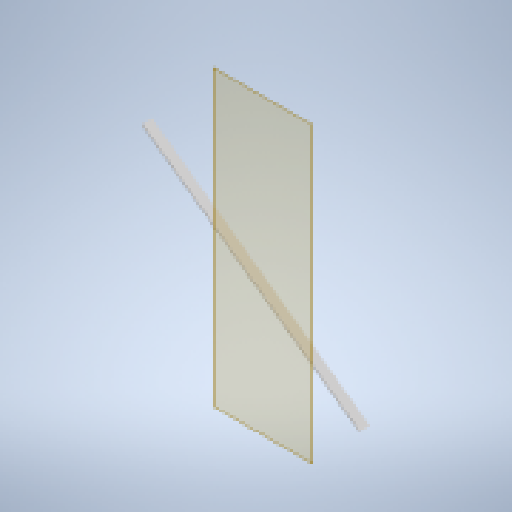
# Autodesk Inventor part: Soportes
Saved by Autodesk Inventor 2024 (Build 280153000, 153)
## iProperties
Created: 2023-08-17
Part Number: Soportes
Material: Genérico
Document SubType Name: Modeling
Designer: sergi
Density: 1 g/cm^3
Appearance: Valor por defecto
Author: sergi
Autodesk Inventor part; units mm, degrees
ref_plane "YZ Plane" through (0, 0, 0) normal (1, 0, 0) x (0, 1, 0)
ref_plane "XZ Plane" through (0, 0, 0) normal (0, 1, 0) x (-1, 0, 0)
ref_plane "XY Plane" through (0, 0, 0) normal (0, 0, 1) x (1, 0, 0)
ref_plane "Plano de trabajo1" through (0, 0, 0) normal (0, 0, 1) x (1, 0, 0)
sketch "Boceto1" plane through (0, 0, 0) normal (0, 0, 1) x (1, 0, 0)
  line L0 (-46.3948, 33.5716) -> (-52.5431, 31.0384) projected
  line L1 (-45.911, 40.2037) -> (-46.3948, 33.5716) projected
  line L2 (-128.559, 100.0083) -> (-45.911, 40.2037) projected
  line L3 (-134.7073, 97.4751) -> (-128.559, 100.0083) projected
  line L4 (-135.1911, 90.843) -> (-134.7073, 97.4751) projected
  line L5 (-52.5431, 31.0384) -> (-135.1911, 90.843) projected
  line L6 (-127.1601, 101.9415) -> (-44.5121, 42.1369) projected
  line L7 (-126.3896, 103.0063) -> (-43.7416, 43.2017) projected
  line L8 (-53.942, 29.1052) -> (-136.59, 88.9098) projected
  line L9 (-137.3604, 87.845) -> (-136.59, 88.9098) projected
  line L10 (-54.7125, 28.0404) -> (-137.3604, 87.845) projected
  line L11 (-126.3896, 103.0063) -> (-127.1601, 101.9415) projected
  line L12 (-136.0968, 89.5913) -> (-53.4489, 29.7866) projected
  line L13 (-45.0053, 41.4554) -> (-127.6532, 101.2601) projected
  line L14 (-127.1601, 101.9415) -> (-131.5092, 100.8886) projected
  line L15 (-136.0968, 89.5913) -> (-135.1911, 90.843) projected
  line L16 (-127.6532, 101.2601) -> (-128.559, 100.0083) projected
  line L17 (-136.59, 88.9098) -> (-136.9497, 93.3701) projected
  line L18 (-136.59, 88.9098) -> (-136.9497, 93.3701) projected
  line L19 (-53.942, 29.1052) -> (-136.59, 88.9098) projected
  line L20 (-49.5929, 30.1581) -> (-53.942, 29.1052) projected
  line L21 (-49.5929, 30.1581) -> (-136.9497, 93.3701) projected
  line L22 (-136.0968, 89.5913) -> (-136.6414, 89.5473)
  line L23 (-53.6337, 29.1798) -> (-136.8536, 89.3983)
  line L24 (-136.8536, 89.3983) -> (-135.6548, 91.0551)
  line L25 (-54.0299, 28.9836) -> (-136.6779, 88.7883)
  line L26 (-49.5929, 30.1581) -> (-53.942, 29.1052) projected
  line L27 (-54.7125, 28.0404) -> (-53.942, 29.1052) projected
  line L28 (-49.5929, 30.1581) -> (-53.942, 29.1052) projected
  line L29 (-53.4489, 29.7866) -> (-49.0998, 30.8396) projected
  line L30 (-53.4489, 29.7866) -> (-52.5431, 31.0384) projected
  line L31 (-54.0299, 28.9836) -> (-53.6337, 29.1798)
  line L32 (-136.6779, 88.7883) -> (-136.6155, 89.2259)
  point P0 (0, 0)
  dimension "d0" = 0.6
  dimension "d1" = 0.15
  constraints: 12 end point, 4 point on line, 1 parallel, 1 perpendicular
  measures "d0" distance between parallel lines of L12 L23
  measures "d1" distance between parallel lines of L8 L25
extrude "Extrusión1" add sketch "Boceto1" against normal blind 3.85 contours L31 L27 L20 | L20 L8 L17 L23 | L27 L25 L9 L8 | L17 L9 L32
ref_plane "Plano de trabajo2" through (-60.3674, 43.6822, 240.2336) normal (0.5862275, 0.8101465, 0) x (0.2890782, -0.2091789, 0.9341724)
sketch "Boceto2" plane through (0, 0, 0) normal (0, 0, 1) x (1, 0, 0)
  line L0 (-53.6337, 29.1798) -> (-136.6155, 89.2259) projected
  line L1 (-136.6155, 89.2259) -> (-136.6779, 88.7883) projected
  line L2 (-136.6779, 88.7883) -> (-54.0299, 28.9836) projected
  line L3 (-54.0299, 28.9836) -> (-53.6337, 29.1798) projected
  circle A0 centre (-136.6467, 89.0071) radius 0.8
  circle A1 centre (-53.8318, 29.0817) radius 0.8
  point P0 (0, 0)
  point P1 (-54.5749, 29.378)
  point P2 (-54.3456, 29.6949)
  point P3 (-135.9036, 88.7108)
  point P4 (-136.1329, 88.3939)
  dimension "d4" = 1.6
  dimension "d5" = 1.6
  constraints: 2 centre point, 2 midpoint
  measures "d4" diameter of A1
  measures "d5" diameter of A0
extrude "Extrusión2" add sketch "Boceto2" against normal blind 1 contours L0 A1 L2 L3 | L0 L1 L2 A0 picked at (-53.7287, 28.8358) picked at (-136.9085, 89.0577)
mirror "Simetría1" about plane through (-60.3674, 43.6822, 240.2336) normal (0.5862275, 0.8101465, 0) of "Extrusión1", "Extrusión2"
